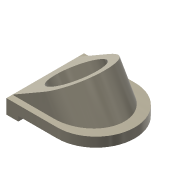
# Autodesk Inventor part: bevelwasher
Saved by Autodesk Inventor 2022 Beta2 (Build 260130000, 130) ContinuousBuild 0
## iProperties
Created: 2008-01-02
Part Number: bevelwasher
Document SubType Name: Modeling
Designer: jmacmillan
Density: 1 g/cm^3
Material: Generic
Appearance: Light Beige
Author: jmacmillan
Autodesk Inventor part; units mm, degrees
ref_plane "YZ Plane" through (0, 0, 0) normal (1, 0, 0) x (0, 1, 0)
ref_plane "XZ Plane" through (0, 0, 0) normal (0, 1, 0) x (-1, 0, 0)
sketch "Sketch1" plane through (0, 0, 0) normal (0, 0, 1) x (1, 0, 0)
  line L0 (0, 91) -> (0, -91) projected
  line L1 (-30, 0) -> (180, 0) projected
  line L2 (0, -65) -> (85, -65)
  arc A0 (85, -65) -> (85, 65) centre (85, 0) ccw
  line L3 (85, 65) -> (0, 65)
  line L4 (0, -65) -> (0, 65)
  dimension "d0" = 65
  dimension "d1" = 85
  constraints: 6 end point, 3 point on line, 2 point on circle, 2 tangent, 1 centre point, 1 collinear, 1 parallel
  measures "d0" distance between parallel lines of L1 L3
  measures "d1" distance of L2.start L2.end
extrude "Extrusion1" add sketch "Sketch1" against normal blind 16
ref_plane "Angular Sketch Plane" through (0, 65, 0) normal (-0.5, 0, 0.8660254) x (0, -1, 0)
sketch "Sketch3" plane through (0, 65, 0) normal (-0.5, 0, 0.8660254) x (0, -1, 0)
  line L0 (0, 0) -> (130, 0) projected
  line L1 (65, -41.3308) -> (65, 191.9846) projected
  line L2 (10, 0) -> (120, 0)
  line L3 (120, 60) -> (120, 0)
  arc A0 (120, 60) -> (10, 60) centre (65, 60) ccw
  line L4 (10, 60) -> (10, 0)
  dimension "d21" = 55
  dimension "d22" = 60
  constraints: 6 end point, 2 point on circle, 2 point on line, 2 tangent, 1 centre point, 1 parallel, 1 perpendicular, 1 other
  measures "d21" radius of A0
  measures "d22" distance from line of A0.centre L0
extrude "Extrusion3" add sketch "Sketch3" against normal up to surface surface through (63.8648, 0, 0) normal (0, 0, 1)
hole "Hole2" at (51.9615, 0, 30) direction (0.5, 0, -0.8660254) diameter 80 end through all
sketch "Sketch4" plane through (0, 0, -16) normal (0, 0, -1) x (-1, 0, 0)
  line L0 (0, -65) -> (-85, -65) projected
  line L1 (0, 65) -> (-20, 65)
  line L2 (-20, 65) -> (-20, -65)
  line L3 (-20, -65) -> (0, -65)
  line L4 (0, -65) -> (0, 65)
  dimension "d34" = 20
  constraints: 8 end point, 2 parallel, 1 horizontal, 1 perpendicular, 1 point on line
  measures "d34" distance of L1.start L1.end
extrude "Extrusion4" add sketch "Sketch4" along normal blind 8
body "Solid1"
